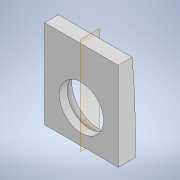
# Autodesk Inventor part: gasVent02
Saved by Autodesk Inventor 2021.1 (Build 251245000, 245)
## iProperties
Created: 2020-08-29
Part Number: gasVent02
Material: Generic
Document SubType Name: Modeling
Designer: robst
Density: 1 g/cm^3
Appearance: Default
Author: robst
Autodesk Inventor part; units mm, degrees
ref_plane "XZ Plane" through (0, 0, 0) normal (0, 1, 0) x (-1, 0, 0)
sketch "Sketch1" plane through (0, 0, 0) normal (1, 0, 0) x (0, 1, 0)
  line L0 (0, 0) -> (0, 12.7)
  line L1 (0, 0) -> (-101.6, 0) construction
  arc A0 (-101.6, 0) -> (0, 0) centre (-50.8, 556.4861) ccw
  line L2 (-50.8, -2.3139) -> (-50.8, 0) construction
  line L3 (0, 12.7) -> (101.6, 12.7) construction
  arc A1 (0, 12.7) -> (101.6, 12.7) centre (50.8, 569.1861) ccw
  line L4 (0, 12.7) -> (-60.96, 12.7)
  line L5 (-60.96, 12.7) -> (-60.96, -2.2215)
  dimension "d0" = 12.7
  dimension "d1" = 101.6
  dimension "d5" = 558.8
  dimension "d6" = 101.6
  dimension "d7" = 558.8
  dimension "d8" = 60.96
  dimension "d24" = 14.9215
  constraints: 12 end point, 6 point on circle, 3 horizontal, 2 centre point, 1 midpoint, 1 perpendicular, 1 vertical
  measures "d0" distance of L0.start L0.end
  measures "d1" distance of L0.start L1.end
  measures "d5" radius of A0
  measures "d6" distance of L0.end L3.end
  measures "d7" radius of A1
  measures "d8" distance of L0.end L4.end
  measures "d24" distance of L4.end L5.end
extrude "Extrusion1" add sketch "Sketch1" along normal mid plane 50.8
sketch "Sketch2" plane through (-25.4, -60.96, 12.7) normal (0, 0, 1) x (1, 0, 0)
  line L0 (25.4, 60.96) -> (25.4, 0) construction
  line L1 (0, 0) -> (50.8, 0) construction
  circle A0 centre (25.4, 22.86) radius 15.24
  line L2 (0, 60.96) -> (50.8, 60.96) projected
  dimension "d11" = 30.48
  dimension "d12" = 38.1
  constraints: 2 end point, 1 centre point, 1 midpoint, 1 point on line
  measures "d11" diameter of A0
  measures "d12" distance from line of A0.centre L2
extrude "Extrusion2" cut sketch "Sketch2" against normal through all
ref_plane "Work Plane2" through (0, -50.8, -2.3139) normal (0, 0, 1) x (1, 0, 0)
sketch "Sketch4" plane through (0, -50.8, -2.3139) normal (0, 0, 1) x (1, 0, 0)
  line L0 (25.4, -10.16) -> (25.4, 50.8) construction
  line L1 (25.4, 46.355) -> (-26.8216, 46.355) construction
  line L2 (-25.4, 50.8) -> (25.4, 50.8) construction
  spline S0 degree 2 poles (21.4174, 43.993) (21.368, 43.9714) (21.1797, 43.9035) (21.0593, 43.8757) knots 0 0 0 1 2 2 2
  spline S1 degree 2 poles (21.0593, 43.8757) (20.9265, 43.8418) (20.7011, 43.8016) (20.5684, 43.8016) knots 0 0 0 1 2 2 2
  spline S2 degree 2 poles (20.5684, 43.8016) (20.3461, 43.8016) (20.0373, 43.9189) (19.9509, 44.0239) knots 0 0 0 1 2 2 2
  spline S3 degree 2 poles (19.9509, 44.0239) (19.8675, 44.1289) (19.8027, 44.4037) (19.8027, 44.5797) knots 0 0 0 1 2 2 2
  line L3 (19.8027, 44.5797) -> (19.8027, 44.8298)
  spline S4 degree 2 poles (19.8027, 44.8298) (19.9972, 44.66) (20.3708, 44.4994) (20.6517, 44.4994) knots 0 0 0 1 2 2 2
  spline S5 degree 2 poles (20.6517, 44.4994) (21.1396, 44.4994) (21.7169, 45.225) (21.7169, 45.9073) knots 0 0 0 1 2 2 2
  spline S6 degree 2 poles (21.7169, 45.9073) (21.7169, 46.2624) (21.5162, 46.812) (21.3495, 47.0065) knots 0 0 0 1 2 2 2
  spline S7 degree 2 poles (21.3495, 47.0065) (21.189, 47.1886) (20.7474, 47.3893) (20.5128, 47.3893) knots 0 0 0 1 2 2 2
  spline S8 degree 2 poles (20.5128, 47.3893) (20.2905, 47.3893) (19.9663, 47.2843) (19.8027, 47.1886) knots 0 0 0 1 2 2 2
  line L4 (19.8027, 47.1886) -> (19.7749, 47.309)
  line L5 (19.7749, 47.309) -> (19.321, 47.309)
  line L6 (19.321, 47.309) -> (19.321, 44.7773)
  spline S9 degree 2 poles (19.321, 44.7773) (19.321, 44.0486) (19.9539, 43.3694) (20.6054, 43.3694) knots 0 0 0 1 2 2 2
  spline S10 degree 2 poles (20.6054, 43.3694) (20.8154, 43.3694) (21.2538, 43.4373) (21.4421, 43.4929) knots 0 0 0 1 2 2 2
  line L7 (21.4421, 43.4929) -> (21.4421, 43.993)
  line L8 (21.4421, 43.993) -> (21.4174, 43.993)
  line L9 (19.8027, 45.225) -> (19.8027, 46.7965)
  spline S11 degree 2 poles (19.8027, 46.7965) (19.9817, 46.883) (20.2843, 46.9571) (20.4356, 46.9571) knots 0 0 0 1 2 2 2
  spline S12 degree 2 poles (20.4356, 46.9571) (20.7999, 46.9571) (21.2198, 46.4198) (21.2198, 45.9166) knots 0 0 0 1 2 2 2
  spline S13 degree 2 poles (21.2198, 45.9166) (21.2198, 45.4411) (20.9018, 44.944) (20.5437, 44.944) knots 0 0 0 1 2 2 2
  spline S14 degree 2 poles (20.5437, 44.944) (20.3553, 44.944) (19.9601, 45.0922) (19.8027, 45.225) knots 0 0 0 1 2 2 2
  line L10 (15.8228, 48.26) -> (17.135, 44.45)
  line L11 (17.135, 44.45) -> (17.6815, 44.45)
  line L12 (17.6815, 44.45) -> (18.9937, 48.26)
  line L13 (18.9937, 48.26) -> (18.4503, 48.26)
  line L14 (18.4503, 48.26) -> (17.3944, 45.0953)
  line L15 (17.3944, 45.0953) -> (16.3385, 48.26)
  line L16 (16.3385, 48.26) -> (15.8228, 48.26)
  line L17 (12.8897, 44.45) -> (12.8897, 47.8092)
  line L18 (12.8897, 47.8092) -> (14.1679, 47.8092)
  line L19 (14.1679, 47.8092) -> (14.1679, 48.26)
  line L20 (14.1679, 48.26) -> (11.1051, 48.26)
  line L21 (11.1051, 48.26) -> (11.1051, 47.8092)
  line L22 (11.1051, 47.8092) -> (12.3833, 47.8092)
  line L23 (12.3833, 47.8092) -> (12.3833, 44.45)
  line L24 (12.3833, 44.45) -> (12.8897, 44.45)
  spline S15 degree 2 poles (8.0207, 47.8247) (7.8046, 47.5715) (7.5637, 46.8305) (7.5637, 46.355) knots 0 0 0 1 2 2 2
  spline S16 degree 2 poles (7.5637, 46.355) (7.5637, 45.8919) (7.7984, 45.1416) (8.0207, 44.8884) knots 0 0 0 1 2 2 2
  spline S17 degree 2 poles (8.0207, 44.8884) (8.2553, 44.6229) (8.8759, 44.3697) (9.2495, 44.3697) knots 0 0 0 1 2 2 2
  spline S18 degree 2 poles (9.2495, 44.3697) (9.6355, 44.3697) (10.253, 44.6322) (10.4783, 44.8884) knots 0 0 0 1 2 2 2
  spline S19 degree 2 poles (10.4783, 44.8884) (10.6976, 45.1416) (10.9322, 45.8857) (10.9322, 46.355) knots 0 0 0 1 2 2 2
  spline S20 degree 2 poles (10.9322, 46.355) (10.9322, 46.8336) (10.6945, 47.5622) (10.4753, 47.8247) knots 0 0 0 1 2 2 2
  spline S21 degree 2 poles (10.4753, 47.8247) (10.253, 48.0778) (9.6324, 48.3403) (9.2495, 48.3403) knots 0 0 0 1 2 2 2
  spline S22 degree 2 poles (9.2495, 48.3403) (8.8605, 48.3403) (8.2368, 48.0686) (8.0207, 47.8247) knots 0 0 0 1 2 2 2
  spline S23 degree 2 poles (8.0917, 46.355) (8.0917, 46.7317) (8.2553, 47.3152) (8.4035, 47.5066) knots 0 0 0 1 2 2 2
  spline S24 degree 2 poles (8.4035, 47.5066) (8.5548, 47.7042) (8.9809, 47.9018) (9.2464, 47.9018) knots 0 0 0 1 2 2 2
  spline S25 degree 2 poles (9.2464, 47.9018) (9.5212, 47.9018) (9.9349, 47.7104) (10.0924, 47.5066) knots 0 0 0 1 2 2 2
  spline S26 degree 2 poles (10.0924, 47.5066) (10.2437, 47.3121) (10.4042, 46.7255) (10.4042, 46.355) knots 0 0 0 1 2 2 2
  spline S27 degree 2 poles (10.4042, 46.355) (10.4042, 45.6047) (9.7744, 44.8082) (9.2464, 44.8082) knots 0 0 0 1 2 2 2
  spline S28 degree 2 poles (9.2464, 44.8082) (8.7185, 44.8082) (8.0917, 45.6047) (8.0917, 46.355) knots 0 0 0 1 2 2 2
  spline S29 degree 2 poles (4.5997, 47.1114) (4.5997, 46.8644) (4.7757, 46.4198) (4.9332, 46.2655) knots 0 0 0 1 2 2 2
  spline S30 degree 2 poles (4.9332, 46.2655) (5.1308, 46.0709) (5.6649, 45.8703) (6.0725, 45.8703) knots 0 0 0 1 2 2 2
  line L25 (6.0725, 45.8703) -> (6.5016, 45.8703)
  line L26 (6.5016, 45.8703) -> (6.5016, 44.45)
  line L27 (6.5016, 44.45) -> (7.008, 44.45)
  line L28 (7.008, 44.45) -> (7.008, 48.26)
  line L29 (7.008, 48.26) -> (6.0508, 48.26)
  spline S31 degree 2 poles (6.0508, 48.26) (5.7112, 48.26) (5.2357, 48.1488) (5.0536, 48.0223) knots 0 0 0 1 2 2 2
  spline S32 degree 2 poles (5.0536, 48.0223) (4.8405, 47.8771) (4.5997, 47.4295) (4.5997, 47.1114) knots 0 0 0 1 2 2 2
  spline S33 degree 2 poles (5.1277, 47.096) (5.1277, 47.2936) (5.2635, 47.5838) (5.4025, 47.6765) knots 0 0 0 1 2 2 2
  spline S34 degree 2 poles (5.4025, 47.6765) (5.5229, 47.7567) (5.844, 47.8216) (6.0817, 47.8216) knots 0 0 0 1 2 2 2
  line L30 (6.0817, 47.8216) -> (6.5016, 47.8216)
  line L31 (6.5016, 47.8216) -> (6.5016, 46.3025)
  line L32 (6.5016, 46.3025) -> (6.1558, 46.3025)
  spline S35 degree 2 poles (6.1558, 46.3025) (5.8471, 46.3025) (5.4673, 46.4013) (5.3438, 46.531) knots 0 0 0 1 2 2 2
  spline S36 degree 2 poles (5.3438, 46.531) (5.2296, 46.6452) (5.1277, 46.9138) (5.1277, 47.096) knots 0 0 0 1 2 2 2
  line L33 (2.6422, 48.4298) -> (4.1335, 43.6225)
  line L34 (4.1335, 43.6225) -> (4.5657, 43.6225)
  line L35 (4.5657, 43.6225) -> (3.0807, 48.4298)
  line L36 (3.0807, 48.4298) -> (2.6422, 48.4298)
  spline S37 degree 2 poles (-0.47, 45.6202) (-0.47, 45.3361) (-0.2539, 44.9008) (-0.0748, 44.7588) knots 0 0 0 1 2 2 2
  spline S38 degree 2 poles (-0.0748, 44.7588) (0.1413, 44.592) (0.6322, 44.45) (1.0213, 44.45) knots 0 0 0 1 2 2 2
  line L37 (1.0213, 44.45) -> (2.1143, 44.45)
  line L38 (2.1143, 44.45) -> (2.1143, 48.26)
  line L39 (2.1143, 48.26) -> (1.1046, 48.26)
  spline S39 degree 2 poles (1.1046, 48.26) (0.6971, 48.26) (0.2895, 48.2075) (0.1043, 48.1056) knots 0 0 0 1 2 2 2
  spline S40 degree 2 poles (0.1043, 48.1056) (-0.1026, 47.9976) (-0.2909, 47.6425) (-0.2909, 47.4017) knots 0 0 0 1 2 2 2
  spline S41 degree 2 poles (-0.2909, 47.4017) (-0.2909, 47.1331) (-0.0069, 46.707) (0.2432, 46.5866) knots 0 0 0 1 2 2 2
  line L40 (0.2432, 46.5866) -> (0.2432, 46.568)
  spline S42 degree 2 poles (0.2432, 46.568) (-0.0964, 46.4754) (-0.47, 45.9845) (-0.47, 45.6202) knots 0 0 0 1 2 2 2
  spline S43 degree 2 poles (0.058, 45.5986) (0.058, 45.8147) (0.1815, 46.0926) (0.3667, 46.1914) knots 0 0 0 1 2 2 2
  spline S44 degree 2 poles (0.3667, 46.1914) (0.4871, 46.2531) (0.7712, 46.2902) (1.0336, 46.2902) knots 0 0 0 1 2 2 2
  line L41 (1.0336, 46.2902) -> (1.6079, 46.2902)
  line L42 (1.6079, 46.2902) -> (1.6079, 44.8823)
  line L43 (1.6079, 44.8823) -> (1.1973, 44.8823)
  spline S45 degree 2 poles (1.1973, 44.8823) (0.8638, 44.8823) (0.481, 44.944) (0.3328, 45.0428) knots 0 0 0 1 2 2 2
  spline S46 degree 2 poles (0.3328, 45.0428) (0.1907, 45.1447) (0.058, 45.3979) (0.058, 45.5986) knots 0 0 0 1 2 2 2
  spline S47 degree 2 poles (0.237, 47.3307) (0.237, 47.4665) (0.3297, 47.6703) (0.4316, 47.7289) knots 0 0 0 1 2 2 2
  spline S48 degree 2 poles (0.4316, 47.7289) (0.5551, 47.7969) (0.8545, 47.8277) (1.1232, 47.8277) knots 0 0 0 1 2 2 2
  line L44 (1.1232, 47.8277) -> (1.6079, 47.8277)
  line L45 (1.6079, 47.8277) -> (1.6079, 46.7132)
  line L46 (1.6079, 46.7132) -> (1.0336, 46.7132)
  spline S49 degree 2 poles (1.0336, 46.7132) (0.7959, 46.7132) (0.5705, 46.7626) (0.4501, 46.8397) knots 0 0 0 1 2 2 2
  spline S50 degree 2 poles (0.4501, 46.8397) (0.3328, 46.9138) (0.237, 47.1516) (0.237, 47.3307) knots 0 0 0 1 2 2 2
  line L47 (-0.5626, 44.45) -> (-1.847, 48.26)
  line L48 (-1.847, 48.26) -> (-2.4707, 48.26)
  line L49 (-2.4707, 48.26) -> (-3.7551, 44.45)
  line L50 (-3.7551, 44.45) -> (-3.221, 44.45)
  line L51 (-3.221, 44.45) -> (-2.8752, 45.5152)
  line L52 (-2.8752, 45.5152) -> (-1.421, 45.5152)
  line L53 (-1.421, 45.5152) -> (-1.0752, 44.45)
  line L54 (-1.0752, 44.45) -> (-0.5626, 44.45)
  line L55 (-2.7362, 45.9474) -> (-2.1465, 47.7413)
  line L56 (-2.1465, 47.7413) -> (-1.5599, 45.9474)
  line L57 (-1.5599, 45.9474) -> (-2.7362, 45.9474)
  spline S51 degree 2 poles (-5.6539, 44.3821) (-5.2834, 44.3821) (-4.6567, 44.6322) (-4.4282, 44.8823) knots 0 0 0 1 2 2 2
  spline S52 degree 2 poles (-4.4282, 44.8823) (-4.1997, 45.1293) (-3.9496, 45.8703) (-3.9496, 46.3519) knots 0 0 0 1 2 2 2
  spline S53 degree 2 poles (-3.9496, 46.3519) (-3.9496, 46.8305) (-4.1935, 47.5406) (-4.4251, 47.803) knots 0 0 0 1 2 2 2
  spline S54 degree 2 poles (-4.4251, 47.803) (-4.6536, 48.0593) (-5.2773, 48.3279) (-5.6632, 48.3279) knots 0 0 0 1 2 2 2
  spline S55 degree 2 poles (-5.6632, 48.3279) (-5.8546, 48.3279) (-6.1912, 48.2724) (-6.3332, 48.2291) knots 0 0 0 1 2 2 2
  spline S56 degree 2 poles (-6.3332, 48.2291) (-6.4567, 48.189) (-6.713, 48.0747) (-6.8396, 48.0068) knots 0 0 0 1 2 2 2
  line L58 (-6.8396, 48.0068) -> (-6.8396, 47.3955)
  line L59 (-6.8396, 47.3955) -> (-6.7994, 47.3955)
  spline S57 degree 2 poles (-6.7994, 47.3955) (-6.7315, 47.4572) (-6.5215, 47.6301) (-6.3702, 47.7135) knots 0 0 0 1 2 2 2
  spline S58 degree 2 poles (-6.3702, 47.7135) (-6.2251, 47.7938) (-5.8824, 47.8957) (-5.6601, 47.8957) knots 0 0 0 1 2 2 2
  spline S59 degree 2 poles (-5.6601, 47.8957) (-5.4162, 47.8957) (-4.9809, 47.695) (-4.8172, 47.5036) knots 0 0 0 1 2 2 2
  spline S60 degree 2 poles (-4.8172, 47.5036) (-4.6567, 47.309) (-4.4776, 46.7193) (-4.4776, 46.3519) knots 0 0 0 1 2 2 2
  spline S61 degree 2 poles (-4.4776, 46.3519) (-4.4776, 45.9598) (-4.6659, 45.3948) (-4.8296, 45.2003) knots 0 0 0 1 2 2 2
  spline S62 degree 2 poles (-4.8296, 45.2003) (-4.9901, 45.0119) (-5.4193, 44.8205) (-5.6601, 44.8205) knots 0 0 0 1 2 2 2
  spline S63 degree 2 poles (-5.6601, 44.8205) (-5.8793, 44.8205) (-6.2529, 44.9286) (-6.398, 45.0088) knots 0 0 0 1 2 2 2
  spline S64 degree 2 poles (-6.398, 45.0088) (-6.537, 45.0891) (-6.7438, 45.2558) (-6.8025, 45.3145) knots 0 0 0 1 2 2 2
  line L60 (-6.8025, 45.3145) -> (-6.8396, 45.3145)
  line L61 (-6.8396, 45.3145) -> (-6.8396, 44.7094)
  spline S65 degree 2 poles (-6.8396, 44.7094) (-6.713, 44.6507) (-6.4907, 44.5426) (-6.3332, 44.4932) knots 0 0 0 1 2 2 2
  spline S66 degree 2 poles (-6.3332, 44.4932) (-6.1665, 44.4376) (-5.8824, 44.3821) (-5.6539, 44.3821) knots 0 0 0 1 2 2 2
  line L62 (-10.0907, 44.45) -> (-9.4331, 44.45)
  line L63 (-9.4331, 44.45) -> (-8.0406, 46.2222)
  line L64 (-8.0406, 46.2222) -> (-7.8183, 45.9721)
  line L65 (-7.8183, 45.9721) -> (-7.8183, 44.45)
  line L66 (-7.8183, 44.45) -> (-7.3119, 44.45)
  line L67 (-7.3119, 44.45) -> (-7.3119, 48.26)
  line L68 (-7.3119, 48.26) -> (-7.8183, 48.26)
  line L69 (-7.8183, 48.26) -> (-7.8183, 46.5094)
  line L70 (-7.8183, 46.5094) -> (-9.3806, 48.26)
  line L71 (-9.3806, 48.26) -> (-9.9981, 48.26)
  line L72 (-9.9981, 48.26) -> (-8.4204, 46.5588)
  line L73 (-8.4204, 46.5588) -> (-10.0907, 44.45)
  spline S67 degree 2 poles (-14.3885, 45.9567) (-14.3885, 45.2404) (-13.7062, 44.3944) (-13.1844, 44.3944) knots 0 0 0 1 2 2 2
  spline S68 degree 2 poles (-13.1844, 44.3944) (-12.9714, 44.3944) (-12.6441, 44.4932) (-12.4743, 44.5951) knots 0 0 0 1 2 2 2
  line L74 (-12.4743, 44.5951) -> (-12.4743, 43.3972)
  line L75 (-12.4743, 43.3972) -> (-11.9926, 43.3972)
  line L76 (-11.9926, 43.3972) -> (-11.9926, 47.309)
  line L77 (-11.9926, 47.309) -> (-12.4743, 47.309)
  line L78 (-12.4743, 47.309) -> (-12.4743, 47.0096)
  spline S69 degree 2 poles (-12.4743, 47.0096) (-12.6534, 47.1732) (-13.0918, 47.3893) (-13.348, 47.3893) knots 0 0 0 1 2 2 2
  spline S70 degree 2 poles (-13.348, 47.3893) (-13.839, 47.3893) (-14.3885, 46.6113) (-14.3885, 45.9567) knots 0 0 0 1 2 2 2
  spline S71 degree 2 poles (-13.8914, 45.9011) (-13.8914, 46.3921) (-13.5796, 46.9324) (-13.2307, 46.9324) knots 0 0 0 1 2 2 2
  spline S72 degree 2 poles (-13.2307, 46.9324) (-13.0269, 46.9324) (-12.6441, 46.7502) (-12.4743, 46.6082) knots 0 0 0 1 2 2 2
  line L79 (-12.4743, 46.6082) -> (-12.4743, 44.9841)
  spline S73 degree 2 poles (-12.4743, 44.9841) (-12.6626, 44.8946) (-12.9312, 44.8267) (-13.1041, 44.8267) knots 0 0 0 1 2 2 2
  spline S74 degree 2 poles (-13.1041, 44.8267) (-13.4777, 44.8267) (-13.8914, 45.3763) (-13.8914, 45.9011) knots 0 0 0 1 2 2 2
  line L80 (-17.6891, 48.26) -> (-16.3769, 44.45)
  line L81 (-16.3769, 44.45) -> (-15.8304, 44.45)
  line L82 (-15.8304, 44.45) -> (-14.5182, 48.26)
  line L83 (-14.5182, 48.26) -> (-15.0616, 48.26)
  line L84 (-15.0616, 48.26) -> (-16.1176, 45.0953)
  line L85 (-16.1176, 45.0953) -> (-17.1735, 48.26)
  line L86 (-17.1735, 48.26) -> (-17.6891, 48.26)
  spline S75 degree 2 poles (-20.3598, 46.355) (-20.3598, 45.3299) (-19.7639, 44.3697) (-19.1433, 44.3697) knots 0 0 0 1 2 2 2
  spline S76 degree 2 poles (-19.1433, 44.3697) (-18.5135, 44.3697) (-17.9238, 45.3485) (-17.9238, 46.3519) knots 0 0 0 1 2 2 2
  spline S77 degree 2 poles (-17.9238, 46.3519) (-17.9238, 47.3831) (-18.5196, 48.3372) (-19.1433, 48.3372) knots 0 0 0 1 2 2 2
  spline S78 degree 2 poles (-19.1433, 48.3372) (-19.7701, 48.3372) (-20.3598, 47.3492) (-20.3598, 46.355) knots 0 0 0 1 2 2 2
  spline S79 degree 2 poles (-19.7052, 45.1941) (-19.7794, 45.3824) (-19.8411, 45.9629) (-19.8411, 46.355) knots 0 0 0 1 2 2 2
  spline S80 degree 2 poles (-19.8411, 46.355) (-19.8411, 46.7471) (-19.7794, 47.3245) (-19.7022, 47.519) knots 0 0 0 1 2 2 2
  spline S81 degree 2 poles (-19.7022, 47.519) (-19.625, 47.7135) (-19.3564, 47.9142) (-19.1433, 47.9142) knots 0 0 0 1 2 2 2
  spline S82 degree 2 poles (-19.1433, 47.9142) (-18.9303, 47.9142) (-18.6555, 47.7135) (-18.5752, 47.5128) knots 0 0 0 1 2 2 2
  spline S83 degree 2 poles (-18.5752, 47.5128) (-18.498, 47.3183) (-18.4425, 46.7255) (-18.4425, 46.3519) knots 0 0 0 1 2 2 2
  spline S84 degree 2 poles (-18.4425, 46.3519) (-18.4425, 45.9505) (-18.4919, 45.4133) (-18.5721, 45.2034) knots 0 0 0 1 2 2 2
  spline S85 degree 2 poles (-18.5721, 45.2034) (-18.6462, 45.0058) (-18.921, 44.7927) (-19.1433, 44.7927) knots 0 0 0 1 2 2 2
  spline S86 degree 2 poles (-19.1433, 44.7927) (-19.3533, 44.7927) (-19.6281, 44.9934) (-19.7052, 45.1941) knots 0 0 0 1 2 2 2
  line L87 (-23.1972, 44.45) -> (-20.8476, 44.45)
  line L88 (-20.8476, 44.45) -> (-20.8476, 44.9903)
  spline S87 degree 2 poles (-20.8476, 44.9903) (-21.1008, 45.2281) (-21.5516, 45.6696) (-21.7677, 45.9073) knots 0 0 0 1 2 2 2
  spline S88 degree 2 poles (-21.7677, 45.9073) (-22.2031, 46.3859) (-22.5211, 46.9602) (-22.5211, 47.2658) knots 0 0 0 1 2 2 2
  spline S89 degree 2 poles (-22.5211, 47.2658) (-22.5211, 47.4264) (-22.4223, 47.6672) (-22.3327, 47.7444) knots 0 0 0 1 2 2 2
  spline S90 degree 2 poles (-22.3327, 47.7444) (-22.2432, 47.8216) (-22.0085, 47.8988) (-21.8665, 47.8988) knots 0 0 0 1 2 2 2
  spline S91 degree 2 poles (-21.8665, 47.8988) (-21.7307, 47.8988) (-21.4528, 47.8308) (-21.3262, 47.7783) knots 0 0 0 1 2 2 2
  spline S92 degree 2 poles (-21.3262, 47.7783) (-21.2181, 47.7351) (-21.0174, 47.6116) (-20.9557, 47.5684) knots 0 0 0 1 2 2 2
  line L89 (-20.9557, 47.5684) -> (-20.9279, 47.5684)
  line L90 (-20.9279, 47.5684) -> (-20.9279, 48.1118)
  spline S93 degree 2 poles (-20.9279, 48.1118) (-21.0854, 48.189) (-21.6504, 48.3403) (-21.9036, 48.3403) knots 0 0 0 1 2 2 2
  spline S94 degree 2 poles (-21.9036, 48.3403) (-22.4377, 48.3403) (-23.0398, 47.7753) (-23.0398, 47.2936) knots 0 0 0 1 2 2 2
  spline S95 degree 2 poles (-23.0398, 47.2936) (-23.0398, 47.0682) (-22.9348, 46.6915) (-22.8422, 46.531) knots 0 0 0 1 2 2 2
  spline S96 degree 2 poles (-22.8422, 46.531) (-22.7495, 46.3643) (-22.4809, 46.037) (-22.3327, 45.8795) knots 0 0 0 1 2 2 2
  spline S97 degree 2 poles (-22.3327, 45.8795) (-22.0919, 45.6171) (-21.5022, 45.0552) (-21.3262, 44.8915) knots 0 0 0 1 2 2 2
  line L91 (-21.3262, 44.8915) -> (-23.1972, 44.8915)
  line L92 (-23.1972, 44.8915) -> (-23.1972, 44.45)
  point P0 (0, 50.8)
  dimension "d18" = 4.445
  constraints: 2 end point, 2 horizontal, 1 point on line
  measures "d18" distance between parallel lines of L1 L2
emboss "Emboss1" sketch "Sketch4" operation cut depth 1.27 direction (0, 0, -1) wrap yes faces at (0.0465, -7.6126, -0.6425)
ref_plane "Work Plane3" through (0, -50.8, -2.3139) normal (0, 0, 1) x (1, 0, 0)
sketch "Sketch5" plane through (0, -50.8, -2.3139) normal (0, 0, 1) x (1, 0, 0)
  circle A0 centre (0, 12.7) radius 15.24 projected
  circle A1 centre (0, 12.7) radius 18.415
  point P0 (0, 50.8)
  dimension "d21" = 3.175
  constraints: 1 centre point, 1 coincident, 1 vertical alignment, 1 other
extrude "Extrusion4" cut sketch "Sketch5" along normal blind 6.35 contours A0 | A1
sketch "Sketch6" plane through (0, 0, 0) normal (1, 0, 0) x (0, 1, 0)
  line L0 (0, 12.7) -> (-60.96, 12.7) projected
  line L1 (0, 0) -> (0, 12.7) projected
  line L2 (-60.96, 12.7) -> (-60.96, -2.2215) projected
  line L3 (0, 12.7) -> (-60.96, 12.7)
  line L4 (-60.96, 12.7) -> (-60.96, 9.525)
  line L5 (-60.96, 9.525) -> (0, 9.525)
  line L6 (0, 9.525) -> (0, 12.7)
  point P0 (0, 9.525)
  dimension "d25" = 3.175
  constraints: 8 end point, 2 parallel, 1 horizontal, 1 perpendicular, 1 point on line
  measures "d25" distance between parallel lines of L0 L5
extrude "Extrusion5" cut sketch "Sketch6" against normal through all both and the other way through all
equation "\"d0\" = sidingDepth"
equation "\"d1\" = sidingHeight"
equation "\"d5\" = radiusOfCurvature"
equation "\"d6\" = sidingHeight"
equation "\"d7\" = radiusOfCurvature"
equation "\"d8\" = partHeight"
equation "\"d9\" = partWidth"
equation "\"d11\" = pipeDiameter"
equation "\"d12\" = pipeCenter"
equation "\"d18\" = textLine"
equation "\"d19\" = textDepth"
equation "\"d21\" = clearanceRingForBackHole"
equation "\"d22\" = clearanceDepth"
equation "\"sidingHeight\" = 101.6"
equation "\"sidingDepth\" = 12.7"
equation "\"radiusOfCurvature\" = 558.8"
equation "\"pipeDiameter\" = 30.48"
equation "\"partWidth\" = 50.8"
equation "\"partHeight\" = 60.96"
equation "\"pipeCenter\" = 38.1"
equation "\"clearanceRingForBackHole\" = 3.175"
equation "\"clearanceDepth\" = 6.35"
equation "\"textLine\" = 4.445"
equation "\"textDepth\" = 1.27"
body "Solid1"
